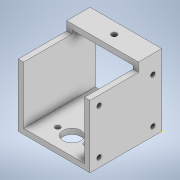
# Autodesk Inventor part: RD006_ギヤボックス左
Saved by Autodesk Inventor 2021.3 (Build 253353000, 353)
## iProperties
Created: 2021-10-14
Part Number: RD006_ギヤボックス左
Material: 一般
Document SubType Name: Modeling
Designer: gilte
Density: 1 g/cm^3
Appearance: 既定
Author: gilte
Autodesk Inventor part; units mm, degrees
ref_plane "YZ Plane" through (0, 0, 0) normal (1, 0, 0) x (0, 1, 0)
ref_plane "XZ Plane" through (0, 0, 0) normal (0, 1, 0) x (-1, 0, 0)
ref_plane "XY Plane" through (0, 0, 0) normal (0, 0, 1) x (1, 0, 0)
sketch "スケッチ1" plane through (0, 0, 0) normal (0, 0, 1) x (1, 0, 0)
  line L0 (0, 0) -> (40, 0)
  line L1 (40, 0) -> (40, 40)
  line L2 (40, 40) -> (0, 40)
  line L3 (0, 40) -> (0, 0)
  line L4 (3, 37) -> (37, 37)
  line L5 (37, 37) -> (37, 3)
  line L6 (37, 3) -> (3, 3)
  line L7 (3, 3) -> (3, 37)
  dimension "d0" = 40
  dimension "d1" = 40
  dimension "d2" = 3
  constraints: 16 end point, 4 parallel, 2 perpendicular, 1 horizontal, 3 other
  measures "d0" distance of L2.end L1.end
  measures "d1" distance of L1.end L0.end
  measures "d2" distance between parallel lines of L2 L4
extrude "押し出し1" add sketch "スケッチ1" along normal blind 40
sketch "スケッチ2" plane through (0, 40, 0) normal (0, 1, 0) x (1, 0, 0)
  line L0 (0, -40) -> (40, -40) projected
  line L1 (0, -40) -> (40, -40)
  line L2 (40, -40) -> (40, -13)
  line L3 (40, -13) -> (0, -13)
  line L4 (0, -13) -> (0, -40)
  point P0 (0, 0)
  dimension "d5" = 40
  dimension "d6" = 27
  constraints: 8 end point, 2 parallel, 1 horizontal, 1 perpendicular
  measures "d5" distance of L3.end L2.end
  measures "d6" distance of L2.end L1.end
extrude "押し出し2" cut sketch "スケッチ2" against normal blind 5
sketch "スケッチ3" plane through (0, 40, 0) normal (0, 1, 0) x (1, 0, 0)
  circle A0 centre (20, -6.5) radius 1.5
  circle A1 centre (20, -30) radius 5
  line L0 (0, -13) -> (40, -13) projected
  line L1 (37, -40) -> (3, -40) projected
  point P0 (0, 0)
  dimension "d9" = 3
  dimension "d10" = 10
  dimension "d11" = 6.5
  dimension "d12" = 10
  constraints: 2 centre point
  measures "d9" diameter of A0
  measures "d10" diameter of A1
  measures "d11" distance from line of L0 A0.centre
  measures "d12" distance from line of L1 A1.centre
extrude "押し出し3" cut sketch "スケッチ3" against normal through all
sketch "スケッチ4" plane through (0, 0, 0) normal (0, -1, 0) x (1, 0, 0)
  circle A0 centre (20, 30) radius 5 projected
  circle A1 centre (20, 6.5) radius 1.5 projected
  line L0 (20, 30) -> (20, 6.5) construction
  line L1 (40, 0) -> (40, 40) construction
  line L2 (0, 40) -> (40, 40) construction
  circle A2 centre (28, 30) radius 1.4 construction
  circle A3 centre (12, 30) radius 1.4 construction
  point P0 (0, 0)
  dimension "d15" = 12
  dimension "d16" = 10
  dimension "d17" = 2.8
  dimension "d18" = 2.8
  constraints: 2 centre point, 2 coincident, 2 end point, 1 symmetric about line, 1 vertical
  measures "d15" distance from line of L1 point (28, 30)
  measures "d16" distance from line of L2 point (28, 30)
  measures "d17" diameter of A2
  measures "d18" diameter of A3
hole "穴1" at (12, 0, 30) at (28, 0, 30) direction (0, 1, 0) diameter 2.8 end through all
sketch "スケッチ5" plane through (40, 0, 0) normal (1, 0, 0) x (0, 0, -1)
  point P0 (0, 0)
sketch "スケッチ6" plane through (40, 0, 0) normal (1, 0, 0) x (0, 0, -1)
  line L0 (0, 0) -> (0, 40) projected
  line L1 (0, 0) -> (-40, 0) projected
  point P0 (-5, 5)
  point P1 (-5, 30)
  point P2 (-35, 5)
  point P3 (-35, 30)
  dimension "d26" = 5
  dimension "d27" = 5
  dimension "d30" = 25
  dimension "d33" = 30
  constraints: 1 horizontal, 1 vertical, 3 other
  measures "d26" distance from line of L0 point (-5, 5)
  measures "d27" distance from line of L1 point (-5, 5)
  measures "d30" distance of point (-5, 5) point (-5, 30)
  measures "d33" distance of point (-5, 5) point (-35, 5)
hole "穴2" at (40, 5, 35) at (40, 30, 35) at (40, 30, 5) at (40, 5, 5) direction (-1, 0, 0) diameter 2.459 depth 3 thread size "M3x0.5" class "6H" standard "ISO Metric profile"
